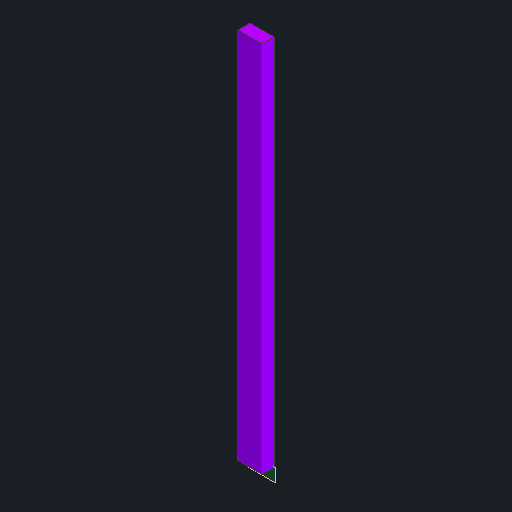
# Autodesk Inventor part: Side piece
Saved by Autodesk Inventor 2027 (Build 310192000, 192)
## iProperties
Created: 2026-05-29
Part Number: Side piece
Material: Generic
Document SubType Name: Modeling
Designer: lucas
Density: 1 g/cm^3
Appearance: Default
Author: lucas
Autodesk Inventor part; units mm, degrees
ref_plane "YZ Plane" through (0, 0, 0) normal (1, 0, 0) x (0, 1, 0)
ref_plane "XZ Plane" through (0, 0, 0) normal (0, 1, 0) x (-1, 0, 0)
ref_plane "XY Plane" through (0, 0, 0) normal (0, 0, 1) x (1, 0, 0)
ref_plane "Work Plane1" through (0, -1676.4, -3657.6) normal (0, 0, -1) x (1, 0, 0)
sketch "Sketch1" plane through (0, -1676.4, -3657.6) normal (0, 0, -1) x (1, 0, 0)
  line L0 (0, -50.8) -> (-101.3938, -50.8) projected
  line L1 (0, -1625.6) -> (-101.3938, -1625.6) projected
  line L2 (0, -50.8) -> (-101.3938, -50.8)
  line L3 (-101.3938, -50.8) -> (-101.3938, -1625.6)
  line L4 (-101.3938, -1625.6) -> (0, -1625.6)
  line L5 (0, -1625.6) -> (0, -50.8)
  point P0 (0, -1676.4)
  point P1 (-101.3938, -50.8)
  constraints: 8 end point, 2 parallel, 1 horizontal, 1 perpendicular
extrude "Extrusion1" add sketch "Sketch1" against normal blind 50.8
body "Solid1"
